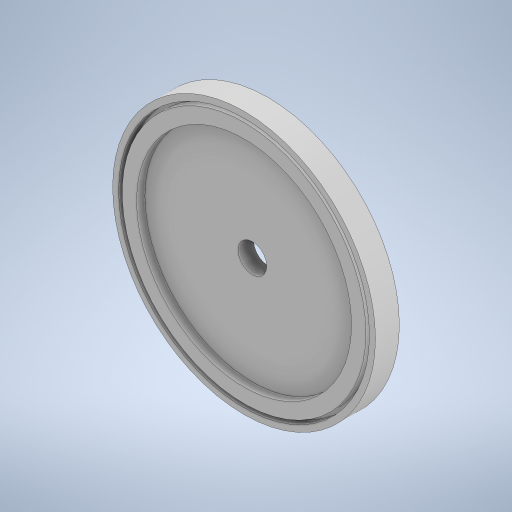
# Autodesk Inventor part: výčko
Saved by Autodesk Inventor 2024.2 (Build 282272000, 272)
## iProperties
Created: 2024-04-30
Part Number: výčko
Material: Všeobecné
Document SubType Name: Modeling
Designer: markoid
Density: 1 g/cm^3
Appearance: Výchozí
Author: markoid
Autodesk Inventor part; units mm, degrees
ref_plane "YZ Plane" through (0, 0, 0) normal (1, 0, 0) x (0, 1, 0)
ref_plane "XZ Plane" through (0, 0, 0) normal (0, 1, 0) x (-1, 0, 0)
ref_plane "XY Plane" through (0, 0, 0) normal (0, 0, 1) x (1, 0, 0)
sketch "Náčrt1" plane through (0, 0, 0) normal (0, 0, 1) x (1, 0, 0)
  line L0 (0, 77) -> (0, -77) projected
  line L1 (-77, 0) -> (77, 0) projected
  circle A0 centre (0, 0) radius 55
  dimension "d0" = 110
  constraints: 1 centre point, 1 coincident
  measures "d0" diameter of A0
extrude "Vysunutí1" add sketch "Náčrt1" along normal blind 10
sketch "Náčrt2" plane through (0, 0, 10) normal (0, 0, 1) x (1, 0, 0)
  circle A0 centre (0, 0) radius 52.5
  circle A1 centre (0, 0) radius 51
  circle A2 centre (0, 0) radius 45
  dimension "d3" = 105
  dimension "d4" = 102
  dimension "d5" = 90
  constraints: 3 centre point, 3 coincident
  measures "d3" diameter of A0
  measures "d4" diameter of A1
  measures "d5" diameter of A2
extrude "Vysunutí2" cut sketch "Náčrt2" against normal blind 3.5
sketch "Náčrt3" plane through (0, 0, 6.5) normal (0, 0, 1) x (1, 0, 0)
  circle A0 centre (0, 0) radius 6
  dimension "d8" = 12
  constraints: 1 centre point, 1 coincident
  measures "d8" diameter of A0
extrude "Vysunutí3" cut sketch "Náčrt3" against normal through all
